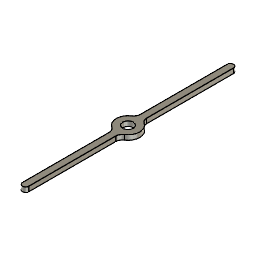
mixer_arm (Autodesk Fusion 360 design; units mm, degrees)
part number: 2026-05-20-12-12-58-237
Autodesk Fusion 360 part; units mm, degrees
sketch "Mixer arm" plane through (0, 0, 0) normal (0, 0, 1) x (1, 0, 0)
  circle A0 centre (0, 0) radius 7.25
  circle A1 centre (0, 0) radius 3.25
  line L0 (-2, 65.25) -> (2, 65.25)
  line L1 (2, 65.25) -> (2, 3.25)
  line L2 (2, 3.25) -> (-2, 3.25)
  line L3 (-2, 3.25) -> (-2, 65.25)
  line L4 (-2, -3.25) -> (2, -3.25)
  line L5 (2, -3.25) -> (2, -65.25)
  line L6 (2, -65.25) -> (-2, -65.25)
  line L7 (-2, -65.25) -> (-2, -3.25)
  line L8 (-2, -7.25) -> (2, -7.25)
  line L9 (-2, 7.25) -> (2, 7.25)
  dimension "d3" = 6.5
  dimension "d5" = 14.5
  dimension "d6" = 2
  dimension "d7" = 2
  dimension "d8" = 2
  dimension "d9" = 2
  dimension "d14" = 58
  dimension "d15" = 58
  constraint coincident A0.centre A1.centre
  constraint concentric A0 A1
  constraint horizontal L0
  constraint vertical L1
  constraint horizontal L2
  constraint vertical L3
  constraint horizontal L4
  constraint vertical L5
  constraint horizontal L6
  constraint vertical L7
  constraint tangent A1 L2
  constraint tangent A1 L4
  constraint coincident L7 L8.start
  constraint coincident L5 L8.end
  constraint perpendicular L5 L8
  constraint tangent A0 L8
  constraint coincident L1 L9.end
  constraint perpendicular L1 L9
  constraint tangent A0 L9
  measures "d3" diameter of A1
  measures "d5" diameter of A0
  measures "d6" distance of A0.centre L1
  measures "d7" distance of A0.centre L3
  measures "d8" distance of A0.centre L7
  measures "d9" distance of A0.centre L5
  measures "d14" distance of L6 L8
  measures "d15" distance of L0 L9
extrude "Extrude1" add sketch "Mixer arm" along normal blind 3 contours A0 A1 L1 L2 L4 L5 | A0 L1 L2 L3 | A0 L1 L9 | A0 L5 L8 | A0 L4 L5 L7 | A0 L3 L9 | L0 L1 L3 L9 | A0 L7 L8 | L5 L6 L7 L8 | A0 A1 L2 L3 L4 L7
fillet "Fillet1" radius 4 4 edges at (2, -6.9687, 1.5) (2, 6.9687, 1.5) (-2, 6.9687, 1.5) (-2, -6.9687, 1.5)
fillet "Fillet2" radius 2 4 edges at (2, 65.25, 1.5) (-2, 65.25, 1.5) (-2, -65.25, 1.5) (2, -65.25, 1.5)
equation "stainless_steel_thickness = 3 mm" comment "The thickness of the 316 stainless steel sheets to laser cut."
equation "hole_diameter = 6.5 mm"
equation "d3 = hole_diameter"
equation "arm_thickness = 4 mm"
equation "d5 = hole_diameter + 2 * arm_thickness"
equation "d6 = arm_thickness / 2"
equation "d7 = arm_thickness / 2"
equation "d8 = arm_thickness / 2"
equation "d9 = arm_thickness / 2"
equation "d10 = stainless_steel_thickness"
equation "arm_length_front = 58 mm"
equation "arm_length_back = 58 mm"
equation "d14 = arm_length_front"
equation "d15 = arm_length_back"
equation "d17 = arm_thickness"
equation "d19 = arm_thickness / 2"
named bodies: "Mixer arm"
